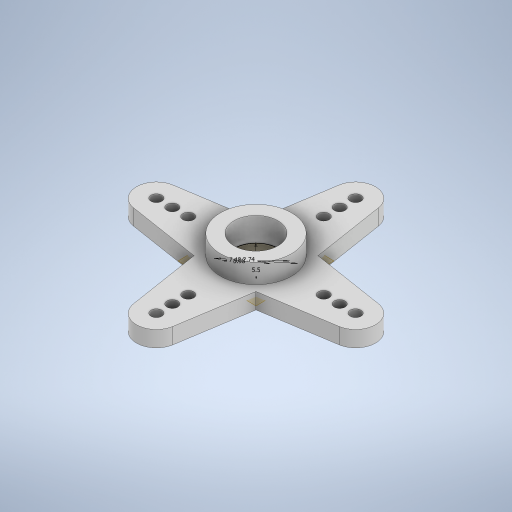
# Autodesk Inventor part: Standard Servo Horn - White Cross
Saved by Autodesk Inventor 2023 (Build 270158000, 158)
## iProperties
Created: 2023-09-05
Part Number: Standard Servo Horn - White Cross
Material: Generic
Document SubType Name: Modeling
Designer: Nate
Density: 1 g/cm^3
Appearance: Default
Author: Nate
Autodesk Inventor part; units mm, degrees
ref_plane "YZ Plane" through (0, 0, 0) normal (1, 0, 0) x (0, 1, 0)
ref_plane "XZ Plane" through (0, 0, 0) normal (0, 1, 0) x (-1, 0, 0)
ref_plane "XY Plane" through (0, 0, 0) normal (0, 0, 1) x (1, 0, 0)
sketch "Sketch1" plane through (0, 0, 0) normal (0, 1, 0) x (-1, 0, 0)
  circle A0 centre (0, 0) radius 3.74
  circle A1 centre (0, 0) radius 4.45
  circle A2 centre (0, 0) radius 8.5
  circle A3 centre (0, 0) radius 10.5
  circle A4 centre (0, 0) radius 12.5
  circle A5 centre (12.5, 0) radius 2.5
  line L0 (0.6942, 4.3955) -> (12.89, 2.4694)
  line L1 (0.6942, -4.3955) -> (12.89, -2.4694)
  circle A6 centre (12.5, 0) radius 0.675
  circle A7 centre (10.5, -0.0001) radius 0.675
  circle A8 centre (8.5, 0.0004) radius 0.675
  line L2 (-4.3955, 0.6942) -> (-2.4694, 12.89)
  circle A9 centre (0, 12.5) radius 2.5
  circle A10 centre (0, 12.5) radius 0.675
  circle A11 centre (0.0001, 10.5) radius 0.675
  circle A12 centre (-0.0004, 8.5) radius 0.675
  line L3 (4.3955, 0.6942) -> (2.4694, 12.89)
  line L4 (-0.6942, -4.3955) -> (-12.89, -2.4694)
  circle A13 centre (-12.5, 0) radius 2.5
  circle A14 centre (-12.5, 0) radius 0.675
  circle A15 centre (-10.5, 0.0001) radius 0.675
  circle A16 centre (-8.5, -0.0004) radius 0.675
  line L5 (-0.6942, 4.3955) -> (-12.89, 2.4694)
  line L6 (4.3955, -0.6942) -> (2.4694, -12.89)
  circle A17 centre (0, -12.5) radius 2.5
  circle A18 centre (0, -12.5) radius 0.675
  circle A19 centre (-0.0001, -10.5) radius 0.675
  circle A20 centre (0.0004, -8.5) radius 0.675
  line L7 (-4.3955, -0.6942) -> (-2.4694, -12.89)
  point P0 (3.8907, 3.8907)
  point P1 (-3.8907, 3.8907)
  point P2 (-3.8907, -3.8907)
  point P3 (3.8907, -3.8907)
  dimension "d5" = 17
  dimension "d6" = 21
  dimension "d7" = 25
  dimension "d3" = 7.48
  dimension "d4" = 8.9
  dimension "d8" = 5
  dimension "d11" = 1.35
  dimension "d12" = 1.35
  dimension "d13" = 1.35
  dimension "d16" = 360
  constraints: 18 centre point, 16 end point, 10 point on circle, 8 coincident, 4 tangent, 1 horizontal alignment, 65 other
  measures "d3" diameter of A0
  measures "d4" diameter of A1
  measures "d8" diameter of A5
  measures "d11" diameter of A6
  measures "d12" diameter of A7
  measures "d13" diameter of A8
extrude "Extrusion1" add sketch "Sketch1" along normal blind 2 contours A1 L3 L0 A2 A8 L1 L6 | A1 L0 L3 | L6 L1 A1 | A1 L5 L2 A2 A12 L3 L0 | L1 L6 A2 A20 L7 L4 A1 | A1 L2 L5 | L0 A3 A5 A7 L1 A2 A8 | A2 A12 L2 A3 A9 A11 L3 | L4 L7 A1 | L6 A3 A17 A19 L7 A2 A20 | A1 L7 L4 A2 A16 L5 L2 | L0 A4 A5 A3 | A3 A9 A4 L3 | A3 A5 A4 L1 | L6 A4 A17 A3 | A2 A16 L4 A3 A13 A15 L5 | A5 A4 A6 A3 A7 | A3 A7 A5 | L0 A5 A4 | A9 A11 A3 | A3 A11 A9 A4 A10 | A4 A9 L3 | A5 A7 A3 | A4 A5 L1 | A17 A4 A18 A3 A19 | A3 A19 A17 | L6 A17 A4 | L2 A4 A9 A3 | A3 A13 A4 L5 | A5 A4 A6 | A4 A10 A9 | L4 A4 A13 A3 | A3 A17 A4 L7 | A17 A4 A18 | A3 A11 A9 | L2 A9 A4 | A13 A15 A3 | A3 A15 A13 A4 A14 | A4 A13 L5 | A3 A15 A13 | L4 A13 A4 | A17 A19 A3 | A4 A17 L7 | A4 A14 A13 picked at (10.283, 0.9379) picked at (0.938, 10.2831) picked at (10.2831, -0.938) picked at (0.9379, -10.283) picked at (-0.9379, 10.283) picked at (-10.2831, 0.938) picked at (-10.283, -0.9379) picked at (-0.938, -10.2831)
extrude "Extrusion2" add sketch "Sketch1" along normal blind 4.44 contours A1
ref_plane "Work Plane2" through (0, 1.44, 0) normal (0, 1, 0) x (1, 0, 0)
sketch "Sketch3" plane through (0, 1.44, 0) normal (0, 1, 0) x (1, 0, 0)
  circle A0 centre (0, 0) radius 1.37
  circle A1 centre (0, 0) radius 2.75
  circle A2 centre (0, 0) radius 2.99
  circle A3 centre (0, 0) radius 3.74
  dimension "d32" = 2.74
  dimension "d33" = 5.5
  dimension "d34" = 5.98
  dimension "d35" = 7.48
  constraints: 4 centre point, 4 coincident
  measures "d32" diameter of A0
  measures "d33" diameter of A1
  measures "d34" diameter of A2
  measures "d35" diameter of A3
extrude "Extrusion6" add sketch "Sketch3" along normal blind 3 and the other way blind 1.94 contours A3
extrude "Extrusion7" add sketch "Sketch3" along normal blind 3 and the other way blind 0.69 contours A2
extrude "Extrusion8" add sketch "Sketch3" against normal blind 0.69 contours A1
body "Solid1"
